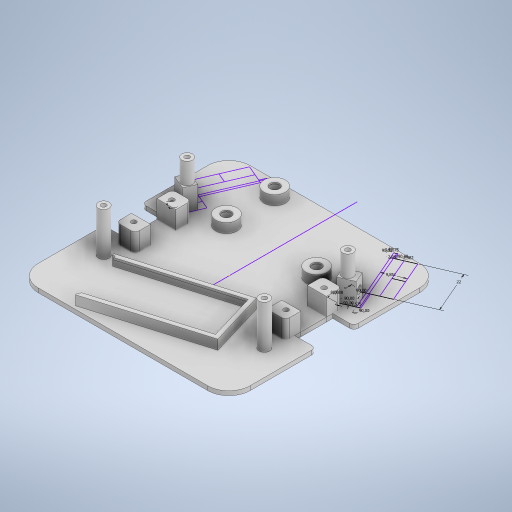
# Autodesk Inventor part: heheheha
Saved by Autodesk Inventor 2023 (Build 270158000, 158)
## iProperties
Created: 2022-12-15
Part Number: heheheha
Material: Ogólny
Document SubType Name: Modeling
Designer: User
Density: 1 g/cm^3
Appearance: Domyślna
Author: User
Autodesk Inventor part; units mm, degrees
ref_plane "YZ Plane" through (0, 0, 0) normal (1, 0, 0) x (0, 1, 0)
ref_plane "XZ Plane" through (0, 0, 0) normal (0, 1, 0) x (-1, 0, 0)
ref_plane "XY Plane" through (0, 0, 0) normal (0, 0, 1) x (1, 0, 0)
sketch "Szkic2" plane through (0, 0, 0) normal (0, 1, 0) x (-1, 0, 0)
  line L0 (50, -50) -> (-50, -50)
  line L1 (50, -50) -> (50, 50)
  line L2 (0, -53.6442) -> (0, 78.3558)
  line L3 (50, 50) -> (-50, 50)
  line L4 (-50, -50) -> (-50, 50)
  line L5 (67.5466, 0) -> (-74.1589, 0)
  line L6 (50, -9) -> (40, -9)
  line L7 (40, -9) -> (40, 9)
  line L8 (40, 9) -> (50, 9)
  line L9 (50, 9) -> (50, -9)
  line L10 (-50, -9) -> (-40, -9)
  line L11 (-40, -9) -> (-40, 9)
  line L12 (-40, 9) -> (-50, 9)
  line L13 (-50, 9) -> (-50, -9)
  line L14 (40, -7.5) -> (31, -7.5)
  line L15 (31, -7.5) -> (31, 7.5)
  line L16 (31, 7.5) -> (40, 7.5)
  line L17 (40, 7.5) -> (40, -7.5)
  line L18 (-40, -7.5) -> (-28.5, -7.5)
  line L19 (-28.5, -7.5) -> (-28.5, 7.5)
  line L20 (-28.5, 7.5) -> (-40, 7.5)
  line L21 (-40, 7.5) -> (-40, -7.5)
  line L22 (31.5, 9) -> (-31.5, 9)
  line L23 (31, 7.5) -> (31, 9)
  line L24 (-28.5, 7.5) -> (-28.5, 9)
  line L25 (31.5, -9) -> (-31.5, -9)
  line L26 (-28.5, -7.5) -> (-28.5, -9)
  line L27 (31, -7.5) -> (31, -9)
  line L28 (40, -11.25) -> (40, -9)
  line L29 (40, 11.25) -> (40, 9)
  line L30 (-40, -11.25) -> (-40, -9)
  line L31 (-40, 11.25) -> (-40, 9)
  circle A0 centre (35.95, -9) radius 1.15
  line L32 (40, -9) -> (40, -7.5)
  line L33 (-40, -9) -> (-40, -7.5)
  line L34 (40, 9) -> (40, 7.5)
  line L35 (-40, 9) -> (-40, 7.5)
  line L36 (40, -9) -> (40, -9)
  line L37 (40, 9) -> (40, 9)
  line L38 (-40, -9) -> (-40, -9)
  line L39 (-40, 9) -> (-40, 9)
  circle A1 centre (35.95, 9) radius 1.15
  circle A2 centre (-35.95, -9) radius 1.15
  circle A3 centre (-35.95, 9) radius 1.15
  line L40 (37.1, -9) -> (37.1, -7.5)
  line L41 (34.8, -9) -> (34.8, -7.5)
  line L42 (40, -14.25) -> (40, -13.75)
  line L43 (37.1, 9) -> (37.1, 7.5)
  line L44 (34.8, 9) -> (34.8, 7.5)
  line L45 (31, 5.5681) -> (31, 11.25)
  line L46 (33, 13.25) -> (38, 13.25)
  line L47 (40, 14.25) -> (40, 13.75)
  circle A4 centre (-35.95, -9) radius 1.15
  line L48 (-37.1, -9) -> (-37.1, -7.5)
  line L49 (-34.8, -9) -> (-34.8, -7.5)
  circle A5 centre (-35.95, 9) radius 1.15
  line L50 (-37.1, 9) -> (-37.1, 7.5)
  line L51 (-34.8, 9) -> (-34.8, 7.5)
  line L52 (-40, -14.25) -> (-40, -13.75)
  line L53 (-31, 9) -> (-31, 11.25)
  line L54 (-40, 14.25) -> (-40, 14.75)
  line L55 (50, -50) -> (50, 50)
  line L56 (50, -50) -> (-50, -50)
  line L57 (50, -9) -> (40, -9)
  line L58 (40, 9) -> (50, 9)
  line L59 (40, 7.5) -> (40, -7.5)
  line L60 (50, -50) -> (-50, -50)
  line L61 (-40, 0) -> (-9.8, 0)
  line L62 (-9.7869, 9) -> (-9.7869, -9)
  line L63 (9.7869, 9) -> (9.7869, -9)
  line L64 (40, -6) -> (31, -6)
  line L65 (40, 6) -> (31, 6)
  line L66 (40, -13.75) -> (40, -9)
  line L67 (31, -5.5681) -> (31, -11.25)
  line L68 (33, -13.25) -> (38, -13.25)
  line L69 (-40, -7.5) -> (-31, -7.5)
  line L70 (-31, 7.5) -> (-40, 7.5)
  circle A6 centre (-35.95, -9) radius 1.15
  circle A7 centre (-35.95, 9) radius 1.15
  line L71 (-37.1, -9) -> (-37.1, -7.5)
  line L72 (-34.8, -9) -> (-34.8, -7.5)
  line L73 (-37.1, 9) -> (-37.1, 7.5)
  line L74 (-34.8, 9) -> (-34.8, 7.5)
  line L75 (-31, 5.5681) -> (-31, 13.25)
  line L76 (-33, 13.25) -> (-38, 13.25)
  line L77 (-40, -6) -> (-31, -6)
  line L78 (-33, -13.25) -> (-38, -13.25)
  line L79 (-31, -5.5681) -> (-31, -11.25)
  arc A8 (38, -13.25) -> (40, -11.25) centre (38, -11.25) ccw
  arc A9 (31, -11.25) -> (33, -13.25) centre (33, -11.25) ccw
  arc A10 (40, 11.25) -> (38, 13.25) centre (38, 11.25) ccw
  arc A11 (33, 13.25) -> (31, 11.25) centre (33, 11.25) ccw
  arc A12 (-31, 11.25) -> (-33, 13.25) centre (-33, 11.25) ccw
  arc A13 (-38, 13.25) -> (-40, 11.25) centre (-38, 11.25) ccw
  arc A14 (-40, -11.25) -> (-38, -13.25) centre (-38, -11.25) ccw
  arc A15 (-33, -13.25) -> (-31, -11.25) centre (-33, -11.25) ccw
  line L80 (-40, 6) -> (-31, 6)
  point P0 (0, 0)
  point P1 (-50, 9)
  point P2 (-34.25, -7.5)
  point P3 (27.1, -10.7133)
  point P4 (31.5, -9)
  point P5 (31.5, -9)
  point P6 (-31.5, 9)
  point P7 (-31.5, 9)
  point P8 (27.1, 10.7133)
  point P9 (40, 7.5)
  point P10 (31, 13.25)
  point P11 (40.0775, 13.25)
  point P12 (-31, -9)
  point P13 (-31, -14.25)
  point P14 (-31, 15.2922)
  point P15 (-34.8, 9)
  point P16 (-37.1, 9)
  point P17 (-37.1, 7.5)
  point P18 (-34.8, 7.5)
  point P19 (-31, 9)
  point P20 (-37.1, -9)
  point P21 (-34.8, -9)
  point P22 (-34.8, -7.5)
  point P23 (-37.1, -7.5)
  point P24 (37.1, 9)
  point P25 (34.8, 9)
  point P26 (34.8, 7.5)
  point P27 (37.1, 7.5)
  point P28 (31, 9)
  point P29 (-50, 0)
  point P30 (31, -13.25)
  point P31 (40.0775, -13.25)
  point P32 (-40.0775, 13.25)
  point P33 (-31, -13.25)
  point P34 (-40.0775, -13.25)
  dimension "d30" = 100
  dimension "d31" = 132
  dimension "d32" = 18
  dimension "d33" = 10
  dimension "d38" = 9
  dimension "d39" = 15
  dimension "d40" = 15
  dimension "d41" = 11.5
  dimension "d42" = 10
  dimension "d44" = 15
  dimension "d47" = 0
  dimension "d50" = 2.3
  dimension "d59" = 2.9
  dimension "d62" = 0.5
  dimension "d68" = 100
  dimension "d69" = 50
  dimension "d70" = 30.2
  dimension "d71" = 1.5
  dimension "d73" = 5.75
  dimension "d74" = 2
  constraints: 158 end point, 51 symmetric about line, 32 point on line, 22 point on circle, 18 tangent, 16 centre point, 14 horizontal, 12 vertical, 9 parallel, 8 perpendicular, 7 equal radius, 7 midpoint, 1 collinear, 68 other
  measures "d30" distance of L0.start L0.end
  measures "d31" distance of L2.start L2.end
  measures "d32" distance of L6.end L7.end
  measures "d33" distance of L6.start L6.end
  measures "d38" distance of L14.start L14.end
  measures "d39" distance of L14.end L15.end
  measures "d40" distance of L20.end L18.start
  measures "d41" distance of L18.start L18.end
  measures "d42" distance of L10.start L10.end
  measures "d44" distance from line of L20 point (-34.25, -7.5)
  measures "d47" distance of L6.end L32.start
  measures "d50" diameter of A0
  measures "d59" distance of L14.start L40.end
  measures "d62" distance of L52.end L52.start
  measures "d68" distance of L0.end L3.end
  measures "d69" distance of point (-50, 0) L3.end
  measures "d70" distance of L61.start L61.end
  measures "d71" distance between parallel lines of L64 L14
  measures "d73" distance between parallel lines of L68 L14
  measures "d74" radius of A8
extrude "Wyciągnięcie proste3" add sketch "Szkic2" along normal blind 10.5 contours L28 A8 L68 A9 L67 L27 L14 L41 A0 L40 L7 | L14 L15 L64 L7 | L11 L18 L48 A2 L49 L79 A15 L78 A14 L30 | L7 L16 L43 A1 L44 L23 L45 A11 L46 A10 L29 | L65 L15 L16 L7 | L40 A0 L41 L14 | L11 L77 L79 L18 | L31 A13 L76 A12 L53 L75 L20 L51 A3 L50 L11 | L11 L20 L75 L80 | L18 L49 A2 L48 | L16 L44 A1 L43 | L50 A3 L51 L20
extrude "Wyciągnięcie proste4" add sketch "Szkic2" along normal blind 2 separate body contours L0 L2 L25 L67 A9 L68 A8 L28 L6 L1 | L0 L4 L10 L30 A14 L78 A15 L79 L25 L2 | L25 L62 L5 L2 | L2 L5 L63 L25 | L28 A8 L68 A9 L67 L27 L14 L41 A0 L40 L7 | L5 L62 L22 L2 | L2 L22 L63 L5 | L63 L5 L15 L27 L25 | L25 L26 L19 L5 L62 | L8 L29 A10 L46 A11 L45 L22 L2 L3 L1 | L7 L64 L15 L5 | L5 L15 L65 L7 | L14 L15 L64 L7 | L11 L18 L48 A2 L49 L79 A15 L78 A14 L30 | L22 L53 A12 L76 A13 L31 L12 L4 L3 L2 | L63 L22 L23 L15 L5 | L5 L19 L24 L22 L62 | L25 L79 L18 L26 | L7 L16 L43 A1 L44 L23 L45 A11 L46 A10 L29 | L65 L15 L16 L7 | L40 A0 L41 L14 | L11 L80 L75 L20 L19 L5 | L5 L19 L18 L79 L77 L11 | L11 L77 L79 L18 | A0 | L31 A13 L76 A12 L53 L75 L20 L51 A3 L50 L11 | L11 L20 L75 L80 | L18 L49 A2 L48 | L24 L20 L75 L22 | L16 L44 A1 L43 | A2 | A1 | L50 A3 L51 L20 | A3
fillet "Zaokrąglenie4" radius 10 4 edges at (-50, 1, -50) (-50, 1, 50) (50, 1, 50) (50, 1, -50)
fillet "Zaokrąglenie5" radius 2 4 edges at (50, 1, 9) (50, 1, -9) (-50, 1, 9) (-50, 1, -9)
sketch "Szkic5" plane through (0, 2, 0) normal (0, 1, 0) x (1, 0, 0)
  line L0 (24.5, 7.6836) -> (-24.5, 7.6836)
  line L1 (-24.5, 7.6836) -> (-24.5, 47.6836)
  line L2 (-24.5, 47.6836) -> (24.5, 47.6836)
  line L3 (24.5, 47.6836) -> (24.5, 7.6836)
  line L4 (0, -42.3954) -> (0, 57.9871)
  line L5 (67.9051, 0) -> (-103.5521, 0)
  circle A0 centre (-21.3, 42.9106) radius 5
  circle A1 centre (-21.3, 20.1106) radius 5
  circle A2 centre (21.3, 20.1106) radius 5
  line L6 (26.631, -32.4148) -> (-23.1992, -47.2793)
  line L7 (-23.1992, -47.2793) -> (-30.3456, -23.3225)
  line L8 (-30.3456, -23.3225) -> (19.4846, -8.458)
  line L9 (19.4846, -8.458) -> (26.631, -32.4148)
  line L10 (27.8751, -33.0872) -> (-23.8716, -48.5234)
  line L11 (-23.8716, -48.5234) -> (-31.5897, -22.6501)
  line L12 (-31.5897, -22.6501) -> (20.157, -7.2139)
  line L13 (20.157, -7.2139) -> (27.8751, -33.0872)
  line L14 (-23.1992, -47.2793) -> (-24.1575, -47.5652)
  line L15 (-30.3456, -23.3225) -> (-31.3038, -23.6083)
  line L16 (26, -27.2838) -> (-27, -27.2838)
  circle A3 centre (-21.3, 42.9106) radius 1.75
  line L17 (-5.4305, -15.8902) -> (1.7159, -39.8471)
  point P0 (0, 0)
  point P1 (0, 7.7958)
  point P2 (0, -14.2703)
  point P3 (0, -13.2268)
  point P4 (0, -41.4025)
  point P5 (0, -40.3589)
  point P6 (0, -27.2838)
  point P7 (3.6487, -26.2263)
  dimension "d75" = 40
  dimension "d76" = 49
  dimension "d78" = 10
  dimension "d79" = 10
  dimension "d86" = 52
  dimension "d87" = 25
  dimension "d88" = 26.631
  dimension "d89" = 1
  dimension "d90" = 1
  dimension "d91" = 1
  dimension "d92" = 1
  dimension "d114" = 3.5
  dimension "d115" = 22.8
  dimension "d123" = 24.5
  dimension "d124" = 42.6
  constraints: 36 end point, 6 parallel, 5 perpendicular, 4 centre point, 4 point on line, 3 horizontal, 3 midpoint, 2 vertical, 1 coincident, 1 symmetric about line
  measures "d75" distance of L2.end L0.start
  measures "d76" distance of L0.start L0.end
  measures "d78" diameter of A0
  measures "d79" diameter of A1
  measures "d86" distance of L7.end L8.end
  measures "d87" distance of L6.end L7.end
  measures "d88" distance from line of L4 L6.start
  measures "d89" distance between parallel lines of L6 L10
  measures "d90" distance between parallel lines of L9 L13
  measures "d91" distance between parallel lines of L7 L11
  measures "d92" distance between parallel lines of L8 L12
  measures "d114" diameter of A3
  measures "d115" distance of A1.centre A0.centre
  measures "d123" distance from line of L4 L0.end
  measures "d124" distance of A2.centre A1.centre
extrude "Wyciągnięcie proste5" add sketch "Szkic5" along normal blind 3.5 contours L12 L13 L10 L4 L6 L9 L8 | L4 L8 L15 L11 L12 | L14 L6 L4 L10 L11 bodies 2
sketch "Szkic7" plane through (0, 5.5, 0) normal (0, 1, 0) x (1, 0, 0)
  line L0 (-31.5897, -22.6501) -> (20.157, -7.2139) projected
  line L1 (-23.8716, -48.5234) -> (-24.1575, -47.5652) projected
  line L2 (19.4846, -8.458) -> (26.631, -32.4148) projected
  line L3 (26.631, -32.4148) -> (-24.1575, -47.5652) projected
  line L4 (-31.3038, -23.6083) -> (19.4846, -8.458) projected
  line L5 (27.8751, -33.0872) -> (-23.8716, -48.5234) projected
  line L6 (20.157, -7.2139) -> (27.8751, -33.0872)
  line L7 (27.8751, -33.0872) -> (-23.8716, -48.5234)
  line L8 (-23.8716, -48.5234) -> (-31.5897, -22.6501)
  line L9 (-31.5897, -22.6501) -> (20.157, -7.2139)
  line L10 (19.4846, -8.458) -> (-31.3038, -23.6083) projected
  line L11 (26.631, -32.4148) -> (19.4846, -8.458) projected
  line L12 (19.4846, -8.458) -> (26.631, -32.4148)
  line L13 (26.631, -32.4148) -> (-23.1992, -47.2793)
  line L14 (-23.1992, -47.2793) -> (-30.3456, -23.3225)
  line L15 (-30.3456, -23.3225) -> (19.4846, -8.458)
  line L16 (18.5263, -8.7439) -> (25.6727, -32.7007)
  line L17 (18.8122, -9.7021) -> (-30.0597, -24.2808)
  line L18 (25.3869, -31.7424) -> (-23.485, -46.321)
  point P0 (0, 0)
  point P1 (22.0995, -20.7223)
  point P2 (-31.5897, -22.6501)
  point P3 (-31.3038, -23.6083)
  point P4 (-30.3456, -23.3225)
  point P5 (-23.1992, -47.2793)
  dimension "d177" = 1
  dimension "d178" = 1
  dimension "d179" = 1
  constraints: 22 end point, 6 perpendicular, 6 point on line, 5 equal length, 1 midpoint
  measures "d177" distance from line of point (22.1, -20.722) L2
  measures "d178" distance between parallel lines of L17 L15
  measures "d179" distance between parallel lines of L13 L18
extrude "Wyciągnięcie proste7" add sketch "Szkic7" along normal blind 1 contours L0 L6 L5 L1 L3 L2 L4 L8 | L4 L16 L17 L14 | L4 L2 L3 L16 | L14 L18 L16 L3 bodies 2
extrude "Wyciągnięcie proste8" add sketch "Szkic5" along normal blind 4.5 contours A2 L3 | L3 A2 | A1 L1 | L1 A1 | A0 L1 L2 | L2 A0 | A0 L1 | A3 picked at (-24.0167, 42.9106) bodies 2
sketch "Szkic8" plane through (-21.3, 6.5, -42.9106) normal (0, 1, 0) x (1, 0, 0)
  circle A0 centre (0, -22.8) radius 5 projected
  circle A1 centre (0, 0) radius 5 projected
  circle A2 centre (42.6, -22.8) radius 5 projected
  point P0 (21.3, -42.9106)
  point P1 (0, -22.8)
  constraints: 3 coincident
hole "Otwór2" at (21.3, 6.5, -20.1106) at (-21.3, 6.5, -42.9106) at (-21.3, 6.5, -20.1106) direction (0, -1, 0) diameter 4 depth 4 counterbore diameter 4.5 counterbore depth 0.6 bodies 2
sketch "Szkic10" plane through (0, 2, 0) normal (0, 1, 0) x (1, 0, 0)
  line L0 (30.6682, 45.4835) -> (39.7138, 49.3848)
  line L1 (39.7138, 49.3848) -> (48.4264, 29.1835)
  line L2 (48.4264, 29.1835) -> (39.3808, 25.2823)
  line L3 (39.3808, 25.2823) -> (30.6682, 45.4835)
  line L4 (32.1145, 46.1073) -> (30.9335, 48.8455)
  line L5 (30.9335, 48.8455) -> (29.4873, 48.2217)
  line L6 (29.4873, 48.2217) -> (30.6682, 45.4835)
  line L7 (35.191, 47.4342) -> (43.9036, 27.2329)
  line L8 (39.5473, 37.3335) -> (44.0701, 39.2842)
  line L9 (44.2937, 17.868) -> (42.8475, 17.2443)
  line L10 (39.3808, 25.2823) -> (42.8475, 17.2443)
  line L11 (44.2937, 17.868) -> (40.827, 25.906)
  line L12 (30.4882, 48.6534) -> (31.6691, 45.9152)
  line L13 (31.6691, 45.9152) -> (43.8484, 17.676)
  line L14 (0, 60.4183) -> (0, -9.1824)
  line L15 (-30.6683, 45.4835) -> (-39.7138, 49.3848)
  line L16 (-39.7138, 49.3848) -> (-48.4264, 29.1835)
  line L17 (-48.4264, 29.1835) -> (-39.3808, 25.2823)
  line L18 (-39.3808, 25.2823) -> (-30.6683, 45.4835)
  line L19 (-32.1145, 46.1073) -> (-30.9335, 48.8455)
  line L20 (-30.9335, 48.8455) -> (-29.4873, 48.2217)
  line L21 (-29.4873, 48.2217) -> (-30.6683, 45.4835)
  line L22 (-35.191, 47.4342) -> (-43.9036, 27.2329)
  line L23 (-39.5473, 37.3335) -> (-44.0701, 39.2842)
  line L24 (-39.3808, 25.2823) -> (-42.8475, 17.2443)
  line L25 (-44.2938, 17.868) -> (-40.8271, 25.906)
  line L26 (-30.4882, 48.6534) -> (-31.6691, 45.9152)
  line L27 (-31.6691, 45.9152) -> (-43.8484, 17.676)
  line L28 (-44.2938, 17.868) -> (-42.8475, 17.2443)
  line L29 (42.8475, 17.2443) -> (36.4198, 14.4721)
  line L30 (38, 13.25) -> (33, 13.25) projected
  line L31 (36.4198, 14.4721) -> (32.9531, 22.5101)
  line L32 (39.3808, 25.2823) -> (32.9531, 22.5101)
  line L33 (-42.8475, 17.2443) -> (-36.4199, 14.4721)
  line L34 (-36.4199, 14.4721) -> (-32.9532, 22.5101)
  line L35 (-39.3808, 25.2823) -> (-32.9532, 22.5101)
  line L36 (-40.1755, 16.0918) -> (-36.7088, 24.1298)
  circle A0 centre (-38.4421, 20.1108) radius 2
  line L37 (34.2417, 19.5224) -> (40.6694, 22.2946)
  line L38 (-34.2417, 19.5224) -> (-40.6694, 22.2946)
  point P0 (0, 0)
  point P1 (-40.3817, 25.714)
  point P2 (-43.8484, 17.676)
  point P3 (40.3817, 25.714)
  dimension "d134" = 9.851
  dimension "d135" = 22
  dimension "d136" = 2.982
  dimension "d138" = 1.575
  dimension "d140" = 90
  dimension "d141" = 90
  dimension "d142" = 2.982
  dimension "d145" = 1.575
  dimension "d146" = 90
  dimension "d147" = 90
  dimension "d148" = 8.038
  dimension "d149" = 1.09
  dimension "d150" = 90
  dimension "d152" = 8.038
  dimension "d153" = 90
  dimension "d155" = 7
  dimension "d159" = 4
  dimension "d171" = 5.5
  constraints: 76 end point, 22 symmetric about line, 13 point on line, 7 perpendicular, 5 midpoint, 3 parallel, 1 centre point, 1 vertical, 1 other
  measures "d134" distance between parallel lines of L1 L3
  measures "d135" distance of L0.end L1.end
  measures "d136" distance of L4.start L4.end
  measures "d138" distance of L4.end L5.end
  measures "d140" angle of L0 L4
  measures "d141" angle of L6 L5
  measures "d142" distance from line of L0 L4.end
  measures "d145" distance of L9.start L9.end
  measures "d146" angle of L10 L2
  measures "d147" angle of L9 L10
  measures "d148" vertical distance of L2.end L9.end
  measures "d149" distance from line of L12 L5.end
  measures "d150" angle of L29 L10
  measures "d152" vertical distance of L31.start L31.end
  measures "d153" angle of L29 L31
  measures "d155" distance of L9.end L29.end
  measures "d159" distance from line of L27 L36.start
  measures "d171" distance from line of L37 L9.end
extrude "Wyciągnięcie proste9" add sketch "Szkic10" along normal blind 10.414 contours L10 L29 L31 L37 | L38 A0 L36 L33 L24 | L38 L36 A0 | L36 A0 L38 L34 L33 | L36 L38 A0 picked at (-38.9603, 19.3109) picked at (-38.6641, 19.1843) bodies 2
sketch "Szkic11" plane through (0, 12.414, 0) normal (0, 1, 0) x (1, 0, 0)
  circle A0 centre (-37.932, 18.2314) radius 2.5
  line L0 (61.8383, -1.4836) -> (-74.9376, -1.4836)
  circle A1 centre (-37.932, -21.1986) radius 2.5
  line L1 (0, -60.0206) -> (0, 63.8525)
  circle A2 centre (37.932, 18.2314) radius 2.5
  circle A3 centre (37.932, -21.1986) radius 2.5
  circle A4 centre (-37.932, -21.1986) radius 1.15
  circle A5 centre (-37.932, 18.2314) radius 1.15
  circle A6 centre (37.932, -21.1986) radius 1.15
  circle A7 centre (37.932, 18.2314) radius 1.15
  circle A8 centre (37.932, 18.2314) radius 2.5
  circle A9 centre (37.932, -21.1986) radius 2.5
  point P0 (0, 0)
  dimension "d163" = 5
  dimension "d170" = 2.3
  dimension "d172" = 39.43
  dimension "d175" = 75.864
  constraints: 10 centre point, 8 symmetric about line, 4 end point, 2 vertical, 1 coincident, 1 horizontal, 8 other
  measures "d163" diameter of A0
  measures "d170" diameter of A4
  measures "d172" distance of A3.centre A2.centre
  measures "d175" distance of A2.centre A0.centre
extrude "Wyciągnięcie proste11" add sketch "Szkic11" along normal blind 10 contours A0 | A2 bodies 2
extrude "Wyciągnięcie proste12" add sketch "Szkic11" along normal blind 10 and the other way blind 10.5 contours A1 | A3 bodies 2
extrude "Wyciągnięcie proste13" add sketch "Szkic11" against normal blind 10.5 contours A6 bodies 2
sketch "Szkic12" plane through (40.6694, 2, -22.2946) normal (0.9182, 0, -0.396) x (-0.396, 0, -0.9182)
  circle A0 centre (-2.75, 5.207) radius 1.75
  line L0 (0, 0) -> (-5.5, 0) projected
  point P0 (-4.3656, -2)
  dimension "d180" = 5.207
  dimension "d181" = 3.5
  constraints: 1 centre point
  measures "d180" distance from line of L0 A0.centre
  measures "d181" diameter of A0
sketch "Szkic13" plane through (-42.8475, 2, -17.2443) normal (-0.9182, 0, -0.396) x (-0.396, 0, 0.9182)
  circle A0 centre (-2.75, 5.207) radius 1.75
  line L0 (0, 0) -> (-5.5, 0) projected
  point P0 (-1.1344, -2)
  dimension "d182" = 5.207
  dimension "d183" = 3.5
  constraints: 1 centre point
  measures "d182" distance from line of L0 A0.centre
  measures "d183" diameter of A0
extrude "Wyciągnięcie proste14" cut sketch "Szkic12" against normal blind 6 bodies 2
extrude "Wyciągnięcie proste15" cut sketch "Szkic13" against normal blind 6 bodies 2
